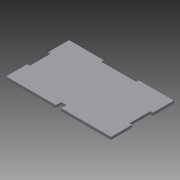
# Autodesk Inventor part: Front
Saved by Autodesk Inventor 2013 (Build 170138000, 138)
## iProperties
Created: 2013-04-20
Part Number: Front
Material: Generic
Document SubType Name: Modeling
Designer: fuji
Density: 1 g/cm^3
Author: fuji
Autodesk Inventor part; units mm, degrees
ref_plane "YZ Plane" through (0, 0, 0) normal (1, 0, 0) x (0, 1, 0)
ref_plane "XZ Plane" through (0, 0, 0) normal (0, 1, 0) x (-1, 0, 0)
ref_plane "XY Plane" through (0, 0, 0) normal (0, 0, 1) x (1, 0, 0)
sketch "Sketch1" plane through (0, 0, 0) normal (0, 0, 1) x (1, 0, 0)
  line L0 (0, 0) -> (127, 0)
  line L1 (127, 0) -> (127, 76.2)
  line L2 (127, 76.2) -> (0, 76.2)
  line L3 (0, 76.2) -> (0, 0)
  dimension "d0" = 127
  dimension "d1" = 76.2
  constraints: 8 end point, 2 parallel, 1 horizontal, 1 perpendicular
  measures "d0" distance of L2.end L1.end
  measures "d1" distance of L1.end L0.end
extrude "Extrusion1" add sketch "Sketch1" along normal blind 3.1496
sketch "Sketch4" plane through (0, 0, 3.1496) normal (0, 0, 1) x (1, 0, 0)
  line L0 (0, 0) -> (127, 0) projected
  line L1 (127, 0) -> (127, 76.2) projected
  line L2 (127, 76.2) -> (0, 76.2) projected
  line L3 (0, 76.2) -> (0, 0) projected
  line L4 (0, 50.8) -> (3.1496, 50.8)
  line L5 (3.1496, 50.8) -> (3.1496, 25.4)
  line L6 (3.1496, 25.4) -> (0, 25.4)
  line L7 (0, 25.4) -> (0, 50.8)
  line L8 (127, 50.8) -> (123.8504, 50.8)
  line L9 (123.8504, 50.8) -> (123.8504, 25.4)
  line L10 (123.8504, 25.4) -> (127, 25.4)
  line L11 (127, 25.4) -> (127, 50.8)
  line L12 (42.3333, 76.2) -> (84.6667, 76.2)
  line L13 (84.6667, 76.2) -> (84.6667, 73.0504)
  line L14 (84.6667, 73.0504) -> (42.3333, 73.0504)
  line L15 (42.3333, 73.0504) -> (42.3333, 76.2)
  dimension "d7" = 3.1496
  dimension "d8" = 25.4
  dimension "d9" = 25.4
  dimension "d10" = 3.1496
  dimension "d11" = 25.4
  dimension "d12" = 25.4
  dimension "d13" = 42.3333
  dimension "d14" = 3.1496
  dimension "d15" = 42.3333
  constraints: 24 end point, 6 parallel, 3 horizontal, 3 perpendicular, 3 point on line
  measures "d7" distance of L5.end L6.end
  measures "d8" distance of L4.end L5.end
  measures "d9" distance between parallel lines of L0 L6
  measures "d10" distance of L10.end L9.end
  measures "d11" distance of L9.end L8.end
  measures "d12" distance between parallel lines of L0 L10
  measures "d13" distance of L13.end L14.end
  measures "d14" distance of L12.end L13.end
  measures "d15" distance between parallel lines of L3 L15
extrude "Extrusion2" cut sketch "Sketch4" against normal blind 3.1496 contours L3 L4 L5 L6 | L10 L9 L8 L1 | L2 L13 L14 L15
sketch "Sketch5" plane through (0, 0, 3.1496) normal (0, 0, 1) x (1, 0, 0)
  line L0 (0, 25.4) -> (0, 0) projected
  line L1 (0, 0) -> (127, 0) projected
  line L2 (60.325, 0) -> (66.675, 0)
  line L3 (66.675, 0) -> (66.675, 6.35)
  line L4 (66.675, 6.35) -> (60.325, 6.35)
  line L5 (60.325, 6.35) -> (60.325, 0)
  dimension "d18" = 6.35
  dimension "d19" = 6.35
  dimension "d20" = 60.325
  constraints: 8 end point, 2 parallel, 1 horizontal, 1 perpendicular, 1 point on line
  measures "d18" distance of L4.end L3.end
  measures "d19" distance of L3.end L2.end
  measures "d20" distance between parallel lines of L5 L0
extrude "Extrusion3" cut sketch "Sketch5" against normal blind 3.1496
equation "\"d0\" = width"
equation "\"d1\" = height"
equation "\"d2\" = thick"
equation "\"d7\" = thick"
equation "\"d8\" = 0.333333 * height"
equation "\"d9\" = 0.333333 * height"
equation "\"d10\" = thick"
equation "\"d11\" = 0.333333 * height"
equation "\"d12\" = 0.333333 * height"
equation "\"d13\" = 0.333333 * width"
equation "\"d14\" = thick"
equation "\"d15\" = 0.333333 * width"
equation "\"d16\" = thick"
equation "\"d21\" = thick"
equation "\"height\" = 76.2"
equation "\"width\" = 127"
equation "\"thick\" = 3.1496"
body "Solid1"
